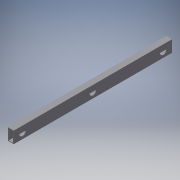
# Autodesk Inventor part: DRL short Angle
Saved by Autodesk Inventor 2018 (Build 220112000, 112)
## iProperties
Created: 2018-01-13
Part Number: DRL short Angle
Material: Generic
Document SubType Name: Modeling
Designer: Orangeracer
Density: 1 g/cm^3
Appearance: Default
Author: Orangeracer
Autodesk Inventor part; units mm, degrees
ref_plane "YZ Plane" through (0, 0, 0) normal (1, 0, 0) x (0, 1, 0)
ref_plane "XZ Plane" through (0, 0, 0) normal (0, 1, 0) x (-1, 0, 0)
ref_plane "XY Plane" through (0, 0, 0) normal (0, 0, 1) x (1, 0, 0)
sketch "Sketch1" plane through (0, 0, 0) normal (0, 0, 1) x (1, 0, 0)
  line L0 (0, 0) -> (25.4, 0)
  line L1 (25.4, 0) -> (25.4, -50.8)
  line L2 (25.4, -50.8) -> (0, -50.8)
  line L3 (0, -50.8) -> (0, 0)
  line L4 (22.225, -3.175) -> (3.175, -3.175)
  line L5 (3.175, -3.175) -> (3.175, -47.625)
  line L6 (3.175, -47.625) -> (22.225, -47.625)
  line L7 (22.225, -47.625) -> (22.225, -3.175)
  dimension "d0" = 25.4
  dimension "d1" = 50.8
  dimension "d2" = 3.175
  constraints: 16 end point, 4 parallel, 2 perpendicular, 1 horizontal, 3 other
  measures "d0" distance of L1.end L2.end
  measures "d1" distance of L0.end L1.end
  measures "d2" distance between parallel lines of L0 L4
extrude "Extrusion1" add sketch "Sketch1" along normal blind 762
sketch "Sketch3" plane through (25.4, -50.8, 0) normal (1, 0, 0) x (0, 0, -1)
  circle A0 centre (-38.1, 25.4) radius 14.2875
  line L0 (0, 50.8) -> (0, 0) projected
  line L1 (0, 50.8) -> (-762, 50.8) projected
  dimension "d13" = 38.1
  dimension "d14" = 25.4
  dimension "d15" = 28.575
  constraints: 1 centre point
  measures "d13" distance from line of L0 A0.centre
  measures "d14" distance from line of L1 A0.centre
  measures "d15" diameter of A0
extrude "Extrusion3" cut sketch "Sketch3" against normal blind 25.4
sketch "Sketch4" plane through (25.4, -50.8, 0) normal (1, 0, 0) x (0, 0, -1)
  circle A0 centre (-723.9, 25.4) radius 14.2875
  circle A1 centre (-381, 25.4) radius 14.2875
  line L0 (-762, 0) -> (-762, 50.8) projected
  line L1 (0, 50.8) -> (-762, 50.8) projected
  circle A2 centre (-38.1, 25.4) radius 14.2875 projected
  dimension "d19" = 38.1
  dimension "d20" = 25.4
  dimension "d21" = 28.575
  dimension "d22" = 25.4
  dimension "d23" = 28.575
  dimension "d26" = 342.9
  dimension "d27" = 342.9
  constraints: 2 centre point
  measures "d19" distance from line of L0 A0.centre
  measures "d20" distance from line of L1 A0.centre
  measures "d21" diameter of A0
  measures "d22" distance from line of L1 A1.centre
  measures "d23" diameter of A1
  measures "d26" distance of A1.centre A0.centre
  measures "d27" distance of A2.centre A1.centre
extrude "Extrusion4" cut sketch "Sketch4" against normal blind 25.4 contours A0 | A1
body "Solid1"
